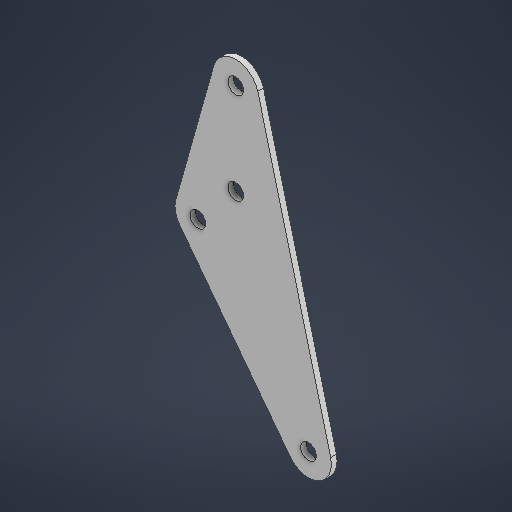
# Autodesk Inventor part: intakesupport
Saved by Autodesk Inventor 2025.2 (Build 292293000, 293)
## iProperties
Created: 2025-03-30
Part Number: intakesupport
Material: Generic
Document SubType Name: Modeling
Designer: roejo
Density: 1 g/cm^3
Appearance: Default
Author: roejo
Autodesk Inventor part; units mm, degrees
ref_plane "YZ Plane" through (0, 0, 0) normal (1, 0, 0) x (0, 1, 0)
ref_plane "XZ Plane" through (0, 0, 0) normal (0, 1, 0) x (-1, 0, 0)
ref_plane "XY Plane" through (0, 0, 0) normal (0, 0, 1) x (1, 0, 0)
sketch "Sketch1" plane through (0, 0, 0) normal (0, 0, 1) x (1, 0, 0)
  circle A0 centre (-4.920941, 38.889745) radius 2.1844
  circle A1 centre (-4.920941, 13.489745) radius 2.1844
  circle A2 centre (-15.45714, 1.56974) radius 2.1844
  circle A3 centre (15.262073, -38.889745) radius 2.1844
  circle A4 centre (15.262073, -38.889745) radius 6.35
  circle A5 centre (-15.45714, 1.56974) radius 6.35
  circle A6 centre (-4.920941, 38.889745) radius 6.35
  line L0 (-21.238079, 4.197144) -> (-11.03537, 40.603294)
  line L1 (1.193489, 40.603294) -> (21.408485, -37.294715)
  line L2 (-20.544521, -2.230399) -> (10.204623, -42.729627)
  point P0 (0, 0)
  dimension "d0" = 12.7
  dimension "d1" = 12.7
  dimension "d2" = 12.7
  constraints: 7 centre point, 6 end point, 6 point on circle, 3 coincident, 3 tangent
  measures "d0" diameter of A4
  measures "d1" diameter of A5
  measures "d2" diameter of A6
sketch "Sketch1 outline for Extrusion1" plane through (0, 0, 0) normal (0, 0, 1) x (1, 0, 0)
  line L0 (-20.544521, -2.230399) -> (10.204623, -42.729627)
  arc A0 (-21.238079, 4.197144) -> (-20.544521, -2.230399) centre (-15.45714, 1.56974) ccw
  arc A1 (10.204623, -42.729627) -> (21.408485, -37.294715) centre (15.262073, -38.889745) ccw
  line L1 (-11.03537, 40.603294) -> (-21.238079, 4.197144)
  line L2 (21.408485, -37.294715) -> (1.193489, 40.603294)
  arc A2 (1.193489, 40.603294) -> (-11.03537, 40.603294) centre (-4.920941, 38.889745) ccw
  circle A3 centre (15.262073, -38.889745) radius 2.1844
  circle A4 centre (-15.45714, 1.56974) radius 2.1844
  circle A5 centre (-4.920941, 13.489745) radius 2.1844
  circle A6 centre (-4.920941, 38.889745) radius 2.1844
extrude "Extrusion1" add sketch "Sketch1 outline for Extrusion1" along normal blind 1.5875
body "Solid1"
